test rotate (Autodesk Fusion 360 design; units mm, degrees)
Autodesk Fusion 360 part; units mm, degrees
note: some values were not read from the file. Set by a fixed rule: which face or edge a step refers to.
sketch "Sketch1" plane through (0, 0, 0) normal (0, 0, 1) x (1, 0, 0)
  circle A0 centre (0, 0) radius 20
  circle A1 centre (0, 18.75) radius 1.25
  line L0 (0, 0) -> (0, 18.75) construction
  circle A2 centre (0, 0) radius 17.5
  dimension "d1" = 40
  dimension "d2" = 2.5
  constraint coincident A0.centre L0.start
  constraint tangent A0 A1
  constraint coincident A1.centre L0.end
  constraint vertical L0
  constraint concentric A0 A2
  constraint tangent A1 A2
  measures "d1" diameter of A0
  measures "d2" diameter of A1
extrude "Extrude1" add sketch "Sketch1" against normal blind 3 contours A2 | A1 | A0
sketch "Sketch2" plane through (0, 0, 0) normal (0, 1, 0) x (1, 0, 0)
  line L0 (0, 0) -> (0, -40)
  dimension "d5" = 40
  constraint coincident L0.start origin
  constraint vertical L0
  measures "d5" distance of L0.start L0.end
ref_plane "WorkPlane1" through (0, 0, 40) normal (0, 0, 1) x (1, 0, 0)
sketch "Sketch3" plane through (0, 0, 40) normal (0, 0, 1) x (1, 0, 0)
  circle A0 centre (0, 18.75) radius 1.25 construction
  line L0 (0, 0) -> (-16.2277, 11.6903) construction
  circle A1 centre (0, 0) radius 20 construction
  circle A2 centre (-15.2135, 10.9596) radius 1.25
  line L1 (0, 0) -> (0, 18.75)
  constraint coincident L0.start A1.centre
  constraint coincident L0.end A1
  constraint coincident L0 A2.centre
  constraint equal A0 A2
  constraint tangent A1 A2
loft "Loft1" add profiles "Sketch1", "Sketch3" section 1 contours A1 section 2
pattern_circular "C-Pattern1" count 8 over 360 about axis through (0, 0, 0) along (0, 0, 1) of "Loft1"
sketch "Sketch4" plane through (0, 0, 40) normal (0, 0, 1) x (-1, 0, 0)
  circle A0 centre (15.2135, -10.9596) radius 1.25
  ellipse E0 centre (3.0079, -18.5072) end of major axis (4.1975, -18.891) minor radius 1.25
  ellipse E1 centre (-10.9596, -15.2135) end of major axis (-10.3899, -16.3261) minor radius 1.25
  ellipse E2 centre (-18.5072, -3.0079) end of major axis (-18.891, -4.1975) minor radius 1.25
  ellipse E3 centre (-15.2135, 10.9596) end of major axis (-16.3261, 10.3899) minor radius 1.25
  ellipse E4 centre (10.9596, 15.2135) end of major axis (10.3899, 16.3261) minor radius 1.25
  ellipse E5 centre (15.2135, -10.9596) end of major axis (16.3261, -10.3899) minor radius 1.25
  circle A1 centre (0, 0) radius 17.5
  circle A2 centre (-3.0079, 18.5072) radius 1.25
  circle A3 centre (18.5072, 3.0079) radius 1.25
  circle A4 centre (0, 0) radius 19.9848
  constraint coincident A1.centre A4.centre
extrude "Extrude3" add sketch "Sketch4" 8 faces at (-11.4978, -15.5446, 40) (14.5616, -10.6848, 40) (18.5589, 2.5794, 40) (10.6848, 14.5616, 40) (-2.3932, 18.7191, 40) (-18.7191, -2.3932, 40) (-15.5446, 11.4978, 40) (3.1683, -18.8413, 40) along normal blind 3 contours A0 E5 A4 | A0 E5 A1 A3 A4 | A0 E5 A4 | A0 E0 E5 A1 A4 | E0 A4 | E0 E1 A1 A4 | E0 A4 | A3 A4 | A3 A4 | E1 A4 | E1 E2 A1 A4 | E4 A1 A3 A4 | E1 A4 | E2 A4 | E2 E3 A1 A4 | E4 A1 A2 A4 | E4 A4 | E4 A4 | E2 A4 | E3 A4 | E3 A1 A2 A4 | A2 A4 | E3 A4 | A2 A4
extrude "Extrude4" cut sketch "Sketch1" against normal blind 24.802 contours A2
